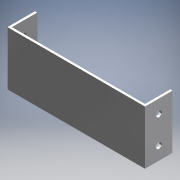
# Autodesk Inventor part: Vertical Support Small
Saved by Autodesk Inventor 2019 (Build 230136000, 136)
## iProperties
Created: 2019-11-04
Part Number: Vertical Support Small
Material: Aluminum 6061
Document SubType Name: Modeling
Designer: Mark
Density: 2.7 g/cm^3
Appearance: Aluminum - Flat
Mass: 44.7334 g
Surface Area: 175.862 cm^2
Volume: 16.5679 cm^3
Author: Mark
Autodesk Inventor part; units mm, degrees
ref_plane "YZ Plane" through (0, 0, 0) normal (1, 0, 0) x (0, 1, 0)
ref_plane "XZ Plane" through (0, 0, 0) normal (0, 1, 0) x (-1, 0, 0)
ref_plane "XY Plane" through (0, 0, 0) normal (0, 0, 1) x (1, 0, 0)
sketch "Sketch1" plane through (0, 0, 0) normal (0, 1, 0) x (-1, 0, 0)
  line L0 (0, 0) -> (125, 0)
  line L1 (125, 0) -> (125, -2)
  line L2 (125, -2) -> (0, -2)
  line L3 (0, -2) -> (0, 0)
  line L4 (0, 0) -> (2, 0)
  line L5 (2, 0) -> (2, -25)
  line L6 (2, -25) -> (0, -25)
  line L7 (0, -25) -> (0, 0)
  line L8 (125, 0) -> (123, 0)
  line L9 (123, 0) -> (123, -25)
  line L10 (123, -25) -> (125, -25)
  line L11 (125, -25) -> (125, 0)
  dimension "d0" = 125
  dimension "d1" = 2
  dimension "d2" = 2
  dimension "d3" = 25
  dimension "d4" = 2
  dimension "d5" = 25
  constraints: 24 end point, 6 parallel, 3 horizontal, 3 perpendicular
  measures "d0" distance of L1.end L2.end
  measures "d1" distance of L0.end L1.end
  measures "d2" distance of L5.end L6.end
  measures "d3" distance of L4.end L5.end
  measures "d4" distance of L10.end L9.end
  measures "d5" distance of L9.end L8.end
extrude "Extrusion1" add sketch "Sketch1" along normal blind 49
sketch "Sketch2" plane through (-125, 0, -25) normal (-1, 0, 0) x (0, 0, 1)
  circle A0 centre (12.5, 12) radius 2.75
  circle A1 centre (12.5, 37) radius 2.75
  line L0 (0, 49) -> (25, 49) projected
  line L1 (0, 0) -> (0, 49) projected
  line L2 (0, 0) -> (25, 0) projected
  dimension "d8" = 5.5
  dimension "d9" = 5.5
  dimension "d10" = 12
  dimension "d11" = 12.5
  dimension "d12" = 12.5
  dimension "d13" = 12
  constraints: 2 centre point
  measures "d8" diameter of A0
  measures "d9" diameter of A1
  measures "d10" distance from line of L0 A1.centre
  measures "d11" distance from line of L1 A1.centre
  measures "d12" distance from line of L1 A0.centre
  measures "d13" distance from line of L2 A0.centre
extrude "Extrusion2" cut sketch "Sketch2" against normal blind 130
body "Solid1"
